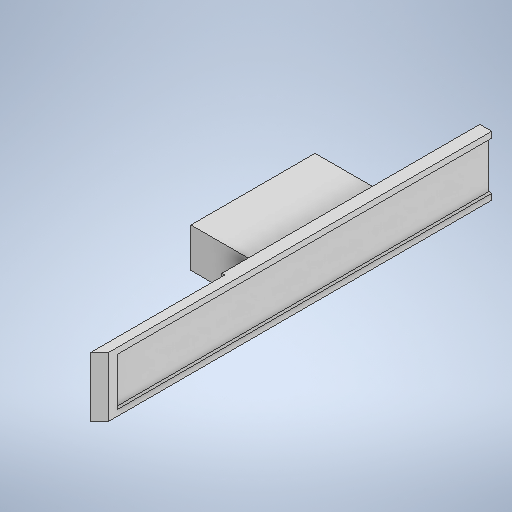
# Autodesk Inventor part: switch_cap
Saved by Autodesk Inventor 2025 (Build 290162000, 162)
## iProperties
Created: 2026-08-05
Part Number: switch_cap
Material: Типовые
Document SubType Name: Modeling
Designer: garin
Density: 1 g/cm^3
Appearance: По умолчанию
Author: garin
Autodesk Inventor part; units mm, degrees
ref_plane "YZ Plane" through (0, 0, 0) normal (1, 0, 0) x (0, 1, 0)
ref_plane "XZ Plane" through (0, 0, 0) normal (0, 1, 0) x (-1, 0, 0)
ref_plane "XY Plane" through (0, 0, 0) normal (0, 0, 1) x (1, 0, 0)
sketch "Эскиз1" plane through (0, 0, 0) normal (1, 0, 0) x (0, 1, 0)
  line L0 (-5, -32.85) -> (5, -32.85)
  line L1 (5, -32.85) -> (5, 32.85)
  line L2 (5, 32.85) -> (-5, 32.85)
  line L3 (-5, 32.85) -> (-5, -32.85)
  line L4 (-5, -32.85) -> (5, 32.85) construction
  line L5 (5, -32.85) -> (-5, 32.85) construction
  line L6 (0, -32.85) -> (0, -16.55) construction
  line L7 (3.3, 4.25) -> (-3.3, 4.25)
  line L8 (-3.3, 4.25) -> (-3.3, -16.55)
  line L9 (-3.3, -16.55) -> (3.3, -16.55)
  line L10 (3.3, -16.55) -> (3.3, 4.25)
  line L11 (5, 32.85) -> (-5, 32.85)
  line L12 (-5, 32.85) -> (-5, 10.35)
  line L13 (-5, 10.35) -> (5, 10.35)
  line L14 (5, 10.35) -> (5, 32.85)
  line L15 (4, 31.85) -> (4, -31.85)
  line L16 (4, -31.85) -> (-4, -31.85) construction
  line L17 (-4, -31.85) -> (-4, 31.85)
  line L18 (-4, 31.85) -> (4, 31.85)
  line L19 (4, -31.85) -> (4, -32.85)
  line L20 (-4, -31.85) -> (-4, -32.85)
  line L21 (4, 31.85) -> (-4, 31.85)
  line L22 (-4, 31.85) -> (-4, 29.85)
  line L23 (-4, 29.85) -> (4, 29.85)
  line L24 (4, 29.85) -> (4, 31.85)
  point P0 (0, 0)
  dimension "d0" = 10
  dimension "d1" = 65.7
  dimension "d2" = 16.3
  dimension "d3" = 6.6
  dimension "d4" = 20.8
  dimension "d5" = 22.5
  dimension "d15" = 1
  dimension "d16" = 2
  constraints: 50 end point, 10 parallel, 7 perpendicular, 4 horizontal, 4 midpoint, 4 point on line, 1 vertical, 3 other
  measures "d0" distance of L2.end L1.end
  measures "d1" distance of L1.end L0.end
  measures "d2" distance of L6.end L6.start
  measures "d3" distance of L9.end L8.end
  measures "d4" distance of L8.end L7.end
  measures "d5" distance of L12.end L11.end
  measures "d15" distance between parallel lines of L1 L15
  measures "d16" distance of L22.end L21.end
extrude "Выдавливание1" add sketch "Эскиз1" along normal blind 2 contours L3 L13 L17 L20 L0 | L20 L17 L13 L15 L19 L0 | L3 L2 L1 L13 L15 L18 L17 | L19 L15 L13 L1 L0 | L17 L23 L15 L13 | L17 L18 L15 L23 | L10 L9 L8 L7
extrude "Выдавливание2" add sketch "Эскиз1" against normal blind 11.3 contours L10 L9 L8 L7
extrude "Выдавливание3" cut sketch "Эскиз1" along normal blind 0.5 contours L3 L2 L1 L13 L15 L18 L17 | L17 L23 L15 L13 | L17 L18 L15 L23
chamfer "Фаска1" distance 1.5 angle 45 1 edges at (2, 0, 32.85)
extrude "Выдавливание4" cut sketch "Эскиз1" against normal blind 0.5 from surface at 2 contours L20 L17 L13 L15 L19 L0 | L17 L23 L15 L13 | L10 L9 L8 L7
